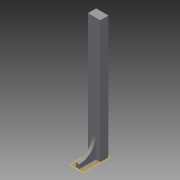
# Autodesk Inventor part: brazo_botella
Saved by Autodesk Inventor 2015 SP1 (Build 190203100, 203)
## iProperties
Created: 2015-07-05
Part Number: brazo_botella
Material: Genérico
Document SubType Name: Modeling
Designer: Javier
Density: 1 g/cm^3
Appearance: Valor por defecto
Author: Javier
Autodesk Inventor part; units mm, degrees
ref_plane "YZ Plane" through (0, 0, 0) normal (1, 0, 0) x (0, 1, 0)
ref_plane "XZ Plane" through (0, 0, 0) normal (0, 1, 0) x (-1, 0, 0)
sketch "Boceto1" plane through (0, 0, 0) normal (0, 0, 1) x (1, 0, 0)
  line L0 (-2, 10) -> (-7.5, 10) projected
  line L1 (7.5, 20) -> (7.5, 10) projected
  line L2 (-7.5, 20) -> (7.5, 20) projected
  line L3 (-7.5, 10) -> (-7.5, 20) projected
  line L4 (7.5, 10) -> (2, 10) projected
  circle A0 centre (0, 15) radius 1.5 projected
  line L5 (-2, 10) -> (-2, -25) projected
  line L6 (-2, -25) -> (2, -25) projected
  line L7 (2, -25) -> (2, 10) projected
  line L8 (2, 10) -> (-2, 10)
  point P0 (0, 0)
  point P1 (-2, -5)
  point P2 (2, -5)
  constraints: 2 end point, 1 collinear
extrude "Extrusión1" add sketch "Boceto1" along normal blind 10 contours L0 L3 L2 L1 L4 L8
sketch "Boceto2" plane through (0, 0, 10) normal (0, 0, 1) x (1, 0, 0)
  line L0 (7.5, 20) -> (-7.5, 20) projected
  line L1 (-7.5, 20) -> (-7.5, 10) projected
  line L2 (7.5, 10) -> (7.5, 20) projected
  line L3 (-7.5, 10) -> (7.5, 10) projected
  point P0 (0, 0)
extrude "Extrusión2" add sketch "Boceto2" along normal blind 220
ref_plane "Plano de trabajo1" through (0, 0, 0) normal (0, 0, 1) x (1, 0, 0)
sketch "Boceto5" plane through (0, 0, 0) normal (0, 0, 1) x (1, 0, 0)
  circle A0 centre (0, -25) radius 60 projected
  line L0 (-2, 10) -> (-7.5, 10) projected
  line L1 (-7.5, 10) -> (-7.5, 20) projected
  line L2 (-7.5, 20) -> (7.5, 20) projected
  line L3 (7.5, 20) -> (7.5, 10) projected
  line L4 (7.5, 10) -> (2, 10) projected
  line L5 (-2, -25) -> (-2, 10) projected
  line L6 (2, 10) -> (2, -25) projected
  line L7 (2, -25) -> (-2, -25) projected
  line L8 (2, 10) -> (-2, 10)
  point P0 (0, 0)
  point P1 (2, -5)
  constraints: 2 end point, 1 collinear
ref_plane "Plano de trabajo2" through (-40, -65, 5) normal (0, 0, 1) x (1, 0, 0)
extrude "Extrusión5" add sketch "Boceto5" along normal up to surface (5 mm away) contours L8 L6 L7 L5
fillet "Empalme1" radius 25 1 edges at (0, 10, 5)
sketch "Boceto6" plane through (-7.5, 20, 0) normal (0, 1, 0) x (1, 0, 0)
  line L0 (15, 0) -> (0, 0) projected
  line L1 (0, 0) -> (0, -230) projected
  line L2 (15, -230) -> (0, -230) projected
  line L3 (15, 0) -> (15, -230) projected
  line L4 (15, -230) -> (0, -230) projected
  line L5 (7.5, -230) -> (7.5, -225)
  line L6 (7.5, -225) -> (7.5, -223)
  circle A0 centre (7.5, -223) radius 2
  point P0 (7.5, 0)
  dimension "d18" = 5
  dimension "d19" = 2
  constraints: 4 end point, 1 coincident, 1 midpoint, 1 point on line, 1 vertical, 1 vertical alignment, 2 other
  measures "d18" distance of L5.start L5.end
  measures "d19" distance of L5.end L6.end
extrude "Extrusión6" cut sketch "Boceto6" against normal blind 5 contours A0
pattern_linear "Patrón rectangular1" count 22 spacing 10 along (0, 0, -1) of "Extrusión6"
